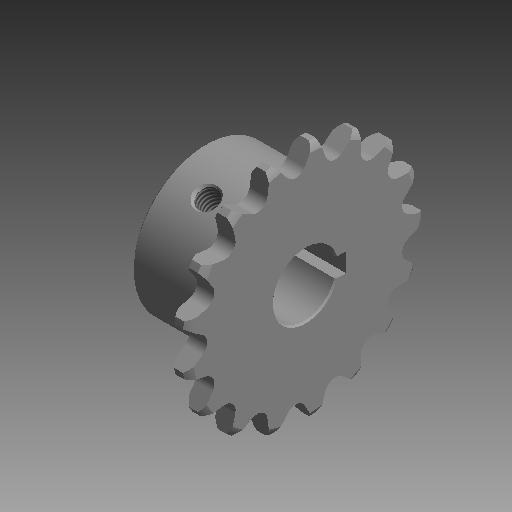
# Autodesk Inventor part: SUSFBN25B17D10_()
Saved by Autodesk Inventor 2019 (Build 230136000, 136)
## iProperties
Category: PARTsolutions
Company: KANA
Part Number: SUSFBN25B17D10_()
Material: 一般
Catalog Web Link: www.cadenas.de
Description: SUSFBN25B-Finished bore
Vendor: KANA
Document SubType Name: Modeling
Designer: partserver
Manufacturer: KANA
Mass: 6.60518 g
Surface Area: 36.7585 cm^2
Volume: 6.60518 cm^3
Density: 1 g/cm^3
Appearance: PSOLRGB-175-175-175
PSOL_IDENT_0: {$CADENAS_DATA\23d-libs\kana\sprockets\chain_no_25\finished_bore_sprocket_steel_stainless\b_type\sus
PSOL_IDENT_1: fbn25b.prj},187 {VTYP=3D},{NB=SUSFBN25B17D10_()},{LINA=SUSFBN25B17D10},{NN=SUSFBN25B},{DATE=02.10.20
PSOL_IDENT_2: 20 05:05:34},{GEOMDATE=02.10.2020 05:05:34},{VERSION=},{LINEID=20},{WBVAR=SD,KS,SURFT},{WBNUMERIC=SD
PSOL_IDENT_3: }  {NB=SUSFBN25B17D10_()},{LINA=SUSFBN25B17D10},{KT=DUMMY},{ORDERNO=SUSFBN25B17D10},{TYPE=SUSFBN25B}
PSOL_IDENT_4: ,{NOT=17},{NOTX=17.000},{DP=34.56},{DO=38},{DC=31.26},{DC2=31.11},{T=2.8},{DR=3.3},{MAT=None},{MATC=
PSOL_IDENT_5: },{SHAPE=C : Cutting type},{SHAPENB=C},{SD=10},{SDX=10},{KS=3 X 1.4},{KSX='3 X 1.4','4 X 1.8'},{M=M4
PSOL_IDENT_6: },{NOTHP=2},{A=6},{SURFT=},{SURFTNB=},{BD=23},{BL=16},{GD=0},{GDX=0},{S=0},{X=0},{VS=0},{SVDEL1=12},
PSOL_IDENT_7: {SVDEL4=4},{SVDEL5=52},{DCX2=1},{B=3},{T2=1.4},{ANGLE=0},{NDM=4},{KDM=3.242},{ONX=},{CAUTION=The too
PSOL_IDENT_8: th profile in the CAD models differ from the actual shape.}
NB: SUSFBN25B17D10_()
NN: SUSFBN25B
NT: Finished bore
NBSYN: SUSFBN25B$NOT.D$SD.$ONX._($SURFT.)
LINA: SUSFBN25B17D10
CATALOG: KANA
TYPE: SUSFBN25B
NOT: 17
DP: 34.56
DO: 38
DC: 31.26
DC2: 31.11
T: 2.8
SHAPE: C : Cutting type
SD: 10
KS: 3 X 1.4
M: M4
NOTHP: 2
A: 6
CAUTION: The tooth profile in the CAD models differ from the actual shape.
SUPPLIER: KANA
ARTICLENO: SUSFBN25B17D10_()
BOMINFO: SUSFBN25B17D10
CREATOR: CADENAS GmbH
Title: SUSFBN25B17D10
Author: Cadenas PARTsolutions
Comments: Finished bore
Autodesk Inventor part; units mm, degrees
sketch "Sketch_1" plane through (0, 0, 0) normal (0, 0, 1) x (1, 0, 0)
  line L0 (16, 0) -> (0, 0)
  line L1 (0, 5.23) -> (0.23, 5)
  line L2 (0.23, 5) -> (15.77, 5)
  line L3 (15.77, 5) -> (16, 5.23)
  line L4 (16, 5.23) -> (16, 11.27)
  line L5 (16, 11.27) -> (15.77, 11.5)
  line L6 (15.77, 11.5) -> (2.8, 11.5)
  line L7 (2.8, 11.5) -> (2.8, 17.8856)
  arc A0 (2.8, 17.8856) -> (2.1, 19) centre (-0.2884, 16.7228) ccw
  line L8 (2.1, 19) -> (0.7, 19)
  arc A1 (0.7, 19) -> (0, 17.8856) centre (3.0884, 16.7228) ccw
  line L9 (0, 17.8856) -> (0, 5.23)
  constraints: 20 end point, 4 point on circle, 2 centre point
revolve "Revolution1" add sketch "Sketch_1" angle 360 about axis through (16, 0, 0) along (1, 0, 0)
sketch "Sketch_7" plane through (1.4, 0, 0) normal (1, 0, 0) x (0, 0, -1)
  circle A0 centre (0, 0) radius 25.3333
  line L0 (-18.9585, 1.2546) -> (-16.4102, -0.1492)
  arc A1 (-16.1582, -2.8687) -> (-16.4102, -0.1492) centre (-17.2063, -1.5944) ccw
  line L1 (-16.1582, -2.8687) -> (-18.4052, -4.7169)
  arc A2 (-18.4052, -4.7169) -> (-18.1315, -5.6787) centre (0, 0) ccw
  line L2 (-18.1315, -5.6787) -> (-15.2481, -6.0671)
  arc A3 (-14.0307, -8.512) -> (-15.2481, -6.0671) centre (-15.4684, -7.7024) ccw
  line L3 (-14.0307, -8.512) -> (-15.4584, -11.0471)
  arc A4 (-15.4584, -11.0471) -> (-14.8558, -11.8451) centre (0, 0) ccw
  line L4 (-14.8558, -11.8451) -> (-12.0268, -11.1657)
  arc A5 (-10.0084, -13.0057) -> (-12.0268, -11.1657) centre (-11.6415, -12.7701) ccw
  line L5 (-10.0084, -13.0057) -> (-10.4239, -15.8853)
  arc A6 (-10.4239, -15.8853) -> (-9.5736, -16.4117) centre (0, 0) ccw
  line L6 (-9.5736, -16.4117) -> (-7.1811, -14.7563)
  arc A7 (-4.6343, -15.7429) -> (-7.1811, -14.7563) centre (-6.2423, -16.1131) ccw
  line L7 (-4.6343, -15.7429) -> (-3.9815, -18.5781)
  arc A8 (-3.9815, -18.5781) -> (-2.9985, -18.7619) centre (0, 0) ccw
  line L8 (-2.9985, -18.7619) -> (-1.3656, -16.3539)
  arc A9 (1.3656, -16.3539) -> (-1.3656, -16.3539) centre (0, -17.28) ccw
  line L9 (1.3656, -16.3539) -> (2.9985, -18.7619)
  arc A10 (2.9985, -18.7619) -> (3.9815, -18.5781) centre (0, 0) ccw
  line L10 (3.9815, -18.5781) -> (4.6343, -15.7429)
  arc A11 (7.1811, -14.7563) -> (4.6343, -15.7429) centre (6.2423, -16.1131) ccw
  line L11 (7.1811, -14.7563) -> (9.5736, -16.4117)
  arc A12 (9.5736, -16.4117) -> (10.4239, -15.8853) centre (0, 0) ccw
  line L12 (10.4239, -15.8853) -> (10.0084, -13.0057)
  arc A13 (12.0268, -11.1657) -> (10.0084, -13.0057) centre (11.6415, -12.7701) ccw
  line L13 (12.0268, -11.1657) -> (14.8558, -11.8451)
  arc A14 (14.8558, -11.8451) -> (15.4584, -11.0471) centre (0, 0) ccw
  line L14 (15.4584, -11.0471) -> (14.0307, -8.512)
  arc A15 (15.2481, -6.0671) -> (14.0307, -8.512) centre (15.4684, -7.7024) ccw
  line L15 (15.2481, -6.0671) -> (18.1315, -5.6787)
  arc A16 (18.1315, -5.6787) -> (18.4052, -4.7169) centre (0, 0) ccw
  line L16 (18.4052, -4.7169) -> (16.1582, -2.8687)
  arc A17 (16.4102, -0.1492) -> (16.1582, -2.8687) centre (17.2063, -1.5944) ccw
  line L17 (16.4102, -0.1492) -> (18.9585, 1.2546)
  arc A18 (18.9585, 1.2546) -> (18.8663, 2.2504) centre (0, 0) ccw
  line L18 (18.8663, 2.2504) -> (16.1033, 3.162)
  arc A19 (15.3559, 5.7889) -> (16.1033, 3.162) centre (16.6203, 4.7289) ccw
  line L19 (15.3559, 5.7889) -> (17.2251, 8.0185)
  arc A20 (17.2251, 8.0185) -> (16.7793, 8.9137) centre (0, 0) ccw
  line L20 (16.7793, 8.9137) -> (13.8737, 8.7657)
  arc A21 (12.2278, 10.9452) -> (13.8737, 8.7657) centre (13.7897, 10.4135) ccw
  line L21 (12.2278, 10.9452) -> (13.1653, 13.6995)
  arc A22 (13.1653, 13.6995) -> (12.4263, 14.3732) centre (0, 0) ccw
  line L22 (12.4263, 14.3732) -> (9.7703, 13.1855)
  arc A23 (7.4482, 14.6233) -> (9.7703, 13.1855) centre (9.0967, 14.6918) ccw
  line L23 (7.4482, 14.6233) -> (7.3275, 17.5302)
  arc A24 (7.3275, 17.5302) -> (6.395, 17.8915) centre (0, 0) ccw
  line L24 (6.395, 17.8915) -> (4.3474, 15.8245)
  arc A25 (1.6627, 16.3264) -> (4.3474, 15.8245) centre (3.1752, 16.9858) ccw
  line L25 (1.6627, 16.3264) -> (0.5, 18.9934)
  arc A26 (0.5, 18.9934) -> (-0.5, 18.9934) centre (0, 0) ccw
  line L26 (-0.5, 18.9934) -> (-1.6627, 16.3264)
  arc A27 (-4.3474, 15.8245) -> (-1.6627, 16.3264) centre (-3.1752, 16.9858) ccw
  line L27 (-4.3474, 15.8245) -> (-6.395, 17.8915)
  arc A28 (-6.395, 17.8915) -> (-7.3275, 17.5302) centre (0, 0) ccw
  line L28 (-7.3275, 17.5302) -> (-7.4482, 14.6233)
  arc A29 (-9.7703, 13.1855) -> (-7.4482, 14.6233) centre (-9.0967, 14.6918) ccw
  line L29 (-9.7703, 13.1855) -> (-12.4263, 14.3732)
  arc A30 (-12.4263, 14.3732) -> (-13.1653, 13.6995) centre (0, 0) ccw
  line L30 (-13.1653, 13.6995) -> (-12.2278, 10.9452)
  arc A31 (-13.8737, 8.7657) -> (-12.2278, 10.9452) centre (-13.7897, 10.4135) ccw
  line L31 (-13.8737, 8.7657) -> (-16.7793, 8.9137)
  arc A32 (-16.7793, 8.9137) -> (-17.2251, 8.0185) centre (0, 0) ccw
  line L32 (-17.2251, 8.0185) -> (-15.3559, 5.7889)
  arc A33 (-16.1033, 3.162) -> (-15.3559, 5.7889) centre (-16.6203, 4.7289) ccw
  line L33 (-16.1033, 3.162) -> (-18.8663, 2.2504)
  arc A34 (-18.8663, 2.2504) -> (-18.9585, 1.2546) centre (0, 0) ccw
  constraints: 68 end point, 68 point on circle, 35 centre point
extrude "Extrusion1" cut sketch "Sketch_7" along normal mid plane 3.2
sketch "Sketch_2" plane through (0, 0, 0) normal (0, 0, 1) x (1, 0, 0)
  line L0 (10, 0) -> (10, 11.5)
  line L1 (10, 11.5) -> (12, 11.5)
  line L2 (12, 11.5) -> (11.621, 11.121)
  line L3 (11.621, 11.121) -> (11.621, 0)
  line L4 (11.621, 0) -> (10, 0)
  line L5 (10, 0) -> (10, 11.5)
  constraints: 12 end point
revolve "Revolution2" cut sketch "Sketch_2" angle 360 about axis through (10, 0, 0) along (0, -1, 0)
thread "Thread1" size "M4x0.7" class "6H" standard "ISO Metric profile" length 4.721
sketch "Sketch_3" plane through (0, 0, 0) normal (0, 0.866, -0.5) x (1, 0, 0)
  line L0 (10, 0) -> (10, 11.5)
  line L1 (10, 11.5) -> (12, 11.5)
  line L2 (12, 11.5) -> (11.621, 11.121)
  line L3 (11.621, 11.121) -> (11.621, 0)
  line L4 (11.621, 0) -> (10, 0)
  line L5 (10, 0) -> (10, 11.5)
  constraints: 12 end point
revolve "Revolution3" cut sketch "Sketch_3" angle 360 about axis through (10, 0, 0) along (0, 0.5, 0.866)
thread "Thread2" size "M4x0.7" class "6H" standard "ISO Metric profile" length 4.721
sketch "Sketch_4" plane through (0, 0, 0) normal (1, 0, 0) x (0, 1, 0)
  line L0 (3.6, 1.5) -> (3.6, -1.5)
  line L1 (3.6, -1.5) -> (6.4, -1.5)
  line L2 (6.4, -1.5) -> (6.4, 1.5)
  line L3 (6.4, 1.5) -> (3.6, 1.5)
  constraints: 8 end point
extrude "Extrusion2" cut sketch "Sketch_4" along normal blind 16
ref_plane "body_XY" through (0, 0, 0) normal (1, 0, 0) x (0, 0, -1)
ref_plane "body_YZ" through (0, 0, 0) normal (0, 0, -1) x (0, 1, 0)
ref_plane "body_ZX" through (0, 0, 0) normal (0, 1, 0) x (1, 0, 0)
body "Solid1"
